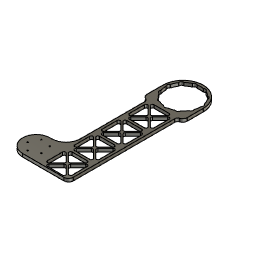
Arm section 1_v10 (Autodesk Fusion 360 design; units mm, degrees)
Autodesk Fusion 360 part; units mm, degrees
sketch "Sketch2" plane through (0, 0, 0) normal (0, 0, 1) x (1, 0, 0)
  line L0 (0, 0) -> (96, 0)
  line L1 (96, 0) -> (96, 96)
  line L2 (96, 96) -> (0, 96)
  line L3 (0, 96) -> (0, 0)
  line L4 (8, 8) -> (88, 8)
  line L5 (88, 8) -> (88, 88)
  line L6 (88, 88) -> (8, 88)
  line L7 (8, 88) -> (8, 8)
  line L8 (8, 88) -> (88, 8) construction
  line L9 (8, 8) -> (88, 88) construction
  line L10 (6.2322, 86.2322) -> (86.2322, 6.2322)
  line L11 (9.7678, 89.7678) -> (89.7678, 9.7678)
  line L12 (9.7678, 6.2322) -> (89.7678, 86.2322)
  line L13 (6.2322, 9.7678) -> (86.2322, 89.7678)
  dimension "d17" = 96
  dimension "d18" = 96
  dimension "d19" = 80
  dimension "d20" = 80
  dimension "d21" = 8
  dimension "d22" = 8
  dimension "d23" = 2.5
  dimension "d24" = -2.5
  dimension "d25" = 2.5
  dimension "d26" = -2.5
  constraint horizontal L0
  constraint vertical L1
  constraint horizontal L2
  constraint vertical L3
  constraint coincident L0.start L3.end
  constraint horizontal L4
  constraint vertical L5
  constraint horizontal L6
  constraint vertical L7
  measures "d17" distance of L0.start L0.end
  measures "d18" distance of L0.start L2.end
  measures "d19" distance of L4.start L4.end
  measures "d20" distance of L4.start L6.end
  measures "d21" distance of L3 L7
  measures "d22" distance of L0 L4
extrude "Extrude2" add sketch "Sketch2" along normal blind 20 contours L0 L1 L2 L3 | L4 L7 L10 L12 L13 | L4 L5 L10 L11 L12 | L10 L11 L12 L13 | L6 L7 L10 L11 L13 | L5 L6 L11 L12 L13 makes body 1
fillet "Fillet1" radius 5 4 edges at (48, 44.4645, 10) (44.4645, 48, 10) (48, 51.5355, 10) (51.5355, 48, 10) on bodies 1
fillet "Fillet1" radius 5 8 edges at (8, 11.5355, 10) (8, 84.4645, 10) (11.5355, 88, 10) (84.4645, 88, 10) (88, 84.4645, 10) (88, 11.5355, 10) (84.4645, 8, 10) (11.5355, 8, 10) on bodies 1
extrude "Extrude3" cut 1 faces at (64, 96, 6.6667) along direction (0, -1, 0) blind 4 on bodies 1 bodies 1
extrude "Extrude4" cut 1 faces at (32, 0, 6.6667) along direction (0, 1, 0) blind 4 on bodies 1 bodies 1
pattern_linear "R-Pattern1" count 4 spacing 88 along (0, 1, 0) of bodies 1 makes body 2 at (93.3333, 127.8689, 0) makes body 3 at (93.3333, 232.1311, 0) makes body 4 at (93.3333, 320.1311, 0)
combine "Combine1" operation add target body 1 tool bodies 2 3 4
sketch "Sketch3" plane through (0, 0, 0) normal (0, 0, 1) x (1, 0, 0)
  line L0 (0, 356) -> (0, 4)
  line L1 (0, 4) -> (-96, 4)
  line L2 (-96, 4) -> (-96, 92)
  line L3 (-96, 92) -> (0, 92)
  line L4 (0, 92) -> (0, 4)
  line L5 (0, 92) -> (-96, 4) construction
  line L6 (-96, 92) -> (0, 4) construction
  circle A0 centre (-48, 48) radius 28 construction
  circle A1 centre (-75.6627, 43.6673) radius 2
  circle A2 centre (-52.4276, 20.3523) radius 2
  circle A3 centre (-23.0737, 35.2455) radius 2
  circle A4 centre (-28.1671, 67.765) radius 2
  circle A5 centre (-60.6689, 72.9699) radius 2
  circle A6 centre (-35.3311, 23.0301) radius 2
  circle A7 centre (-67.8329, 28.235) radius 2
  circle A8 centre (-72.9263, 60.7545) radius 2
  circle A9 centre (-43.5724, 75.6477) radius 2
  circle A10 centre (-20.3373, 52.3327) radius 2
  dimension "d44" = 96
  dimension "d45" = 88
  dimension "d46" = 56
  dimension "d47" = 4
  dimension "d49" = 360
  dimension "d145" = 360
  constraint horizontal L1
  constraint vertical L2
  constraint horizontal L3
  constraint vertical L4
  constraint coincident L0.end L1.start
  constraint midpoint L5 A0.centre
  constraint coincident A0 A1.centre
  measures "d44" distance of L0.end L1.end
  measures "d45" distance of L0.end L3.end
  measures "d46" diameter of A0
  measures "d47" diameter of A1
extrude "Extrude5" add sketch "Sketch3" along normal blind 20 bodies 1
fillet "Fillet2" radius 44 2 edges at (-96, 92, 10) (-96, 4, 10) on bodies 1
fillet "Fillet3" radius 46 1 edges at (0, 92, 10) on bodies 1
fillet "Fillet4" radius 15 1 edges at (96, 4, 10) on bodies 1
extrude "Extrude7" cut 1 faces at (-0.7791, 49.4442, 20) along direction (0, 0, -1) blind 10 on bodies 1 bodies 1
sketch "Sketch6" plane through (0, 0, 0) normal (0, 0, 1) x (1, 0, 0)
  circle A0 centre (48, 436) radius 65
  circle A1 centre (48, 436) radius 80
  line L0 (0, 356) -> (96, 356)
  line L1 (96, 356) -> (128, 356) construction
  line L2 (128, 356) -> (-32, 356)
  line L3 (-32, 356) -> (-32, 516)
  line L4 (-32, 516) -> (128, 516)
  line L5 (128, 516) -> (128, 356)
  point P0 (96, 356)
  point P1 (0, 356)
  dimension "d78" = 130
  dimension "d81" = 160
  dimension "d89" = 80
  dimension "d90" = 32
  dimension "d91" = 160
  dimension "d92" = 160
  constraint concentric A0 A1
  constraint coincident P0 L0.end
  constraint parallel L0 L1
  constraint horizontal L2
  constraint vertical L3
  constraint horizontal L4
  constraint vertical L5
  measures "d78" diameter of A0
  measures "d81" diameter of A1
  measures "d89" distance of A0.centre L0
  measures "d90" distance of P0 L1.end
  measures "d91" distance of L1.end L2.end
  measures "d92" distance of L1.end L4.end
extrude "Extrude8" add sketch "Sketch6" along normal blind 10 contours A1 | A1 L0 L2 L5 | A1 L0 L2 L3 bodies 1
fillet "Fillet6" radius 15 2 edges at (96, 356, 5) (0, 356, 5) on bodies 1
fillet "Fillet6" radius 15 2 edges at (-32, 356, 5) (128, 356, 5) on bodies 1
sketch "Sketch7" plane through (0, 0, 10) normal (0, 0, 1) x (-1, 0, 0)
  arc A0 (-113, -356) -> (-128, -371) centre (-113, -371) ccw
  line L0 (-128, -371) -> (-128, -436)
  arc A1 (-128, -436) -> (32, -436) centre (-48, -436) ccw
  line L1 (32, -436) -> (32, -371)
  arc A2 (32, -371) -> (17, -356) centre (17, -371) ccw
  line L2 (17, -356) -> (15, -356)
  arc A3 (0, -341) -> (15, -356) centre (15, -341) ccw
  line L3 (0, -341) -> (0, -138)
  arc A4 (46, -92) -> (0, -138) centre (46, -138) ccw
  line L4 (46, -92) -> (52, -92)
  arc A5 (52, -92) -> (52, -4) centre (52, -48) ccw
  line L5 (52, -4) -> (-81, -4)
  arc A6 (-81, -4) -> (-96, -19) centre (-81, -19) ccw
  line L6 (-96, -19) -> (-96, -341)
  arc A7 (-111, -356) -> (-96, -341) centre (-111, -341) ccw
  line L7 (-111, -356) -> (-113, -356)
  circle A8 centre (-48, -436) radius 65
  circle A9 centre (23.0737, -35.2455) radius 2
  circle A10 centre (75.6627, -43.6673) radius 2
  circle A11 centre (52.4276, -20.3523) radius 2
  circle A12 centre (60.6689, -72.9699) radius 2
  circle A13 centre (28.1671, -67.765) radius 2
  line L8 (-20.0711, -280.5355) -> (-44.4645, -304.9289)
  arc A14 (-51.5355, -304.9289) -> (-44.4645, -304.9289) centre (-48, -301.3934) ccw
  line L9 (-51.5355, -304.9289) -> (-75.9289, -280.5355)
  arc A15 (-72.3934, -272) -> (-75.9289, -280.5355) centre (-72.3934, -277) ccw
  line L10 (-72.3934, -272) -> (-23.6066, -272)
  arc A16 (-20.0711, -280.5355) -> (-23.6066, -272) centre (-23.6066, -277) ccw
  line L11 (-79.4645, -284.0711) -> (-55.0711, -308.4645)
  arc A17 (-55.0711, -315.5355) -> (-55.0711, -308.4645) centre (-58.6066, -312) ccw
  line L12 (-55.0711, -315.5355) -> (-79.4645, -339.9289)
  arc A18 (-88, -336.3934) -> (-79.4645, -339.9289) centre (-83, -336.3934) ccw
  line L13 (-88, -336.3934) -> (-88, -287.6066)
  arc A19 (-79.4645, -284.0711) -> (-88, -287.6066) centre (-83, -287.6066) ccw
  line L14 (-8, -287.6066) -> (-8, -336.3934)
  arc A20 (-16.5355, -339.9289) -> (-8, -336.3934) centre (-13, -336.3934) ccw
  line L15 (-16.5355, -339.9289) -> (-40.9289, -315.5355)
  arc A21 (-40.9289, -308.4645) -> (-40.9289, -315.5355) centre (-37.3934, -312) ccw
  line L16 (-40.9289, -308.4645) -> (-16.5355, -284.0711)
  arc A22 (-8, -287.6066) -> (-16.5355, -284.0711) centre (-13, -287.6066) ccw
  line L17 (-44.4645, -319.0711) -> (-20.0711, -343.4645)
  arc A23 (-23.6066, -352) -> (-20.0711, -343.4645) centre (-23.6066, -347) ccw
  line L18 (-23.6066, -352) -> (-72.3934, -352)
  arc A24 (-75.9289, -343.4645) -> (-72.3934, -352) centre (-72.3934, -347) ccw
  line L19 (-75.9289, -343.4645) -> (-51.5355, -319.0711)
  arc A25 (-44.4645, -319.0711) -> (-51.5355, -319.0711) centre (-48, -322.6066) ccw
  line L20 (-20.0711, -192.5355) -> (-44.4645, -216.9289)
  arc A26 (-51.5355, -216.9289) -> (-44.4645, -216.9289) centre (-48, -213.3934) ccw
  line L21 (-51.5355, -216.9289) -> (-75.9289, -192.5355)
  arc A27 (-72.3934, -184) -> (-75.9289, -192.5355) centre (-72.3934, -189) ccw
  line L22 (-72.3934, -184) -> (-23.6066, -184)
  arc A28 (-20.0711, -192.5355) -> (-23.6066, -184) centre (-23.6066, -189) ccw
  line L23 (-79.4645, -196.0711) -> (-55.0711, -220.4645)
  arc A29 (-55.0711, -227.5355) -> (-55.0711, -220.4645) centre (-58.6066, -224) ccw
  line L24 (-55.0711, -227.5355) -> (-79.4645, -251.9289)
  arc A30 (-88, -248.3934) -> (-79.4645, -251.9289) centre (-83, -248.3934) ccw
  line L25 (-88, -248.3934) -> (-88, -199.6066)
  arc A31 (-79.4645, -196.0711) -> (-88, -199.6066) centre (-83, -199.6066) ccw
  line L26 (-8, -199.6066) -> (-8, -248.3934)
  arc A32 (-16.5355, -251.9289) -> (-8, -248.3934) centre (-13, -248.3934) ccw
  line L27 (-16.5355, -251.9289) -> (-40.9289, -227.5355)
  arc A33 (-40.9289, -220.4645) -> (-40.9289, -227.5355) centre (-37.3934, -224) ccw
  line L28 (-40.9289, -220.4645) -> (-16.5355, -196.0711)
  arc A34 (-8, -199.6066) -> (-16.5355, -196.0711) centre (-13, -199.6066) ccw
  line L29 (-44.4645, -231.0711) -> (-20.0711, -255.4645)
  arc A35 (-23.6066, -264) -> (-20.0711, -255.4645) centre (-23.6066, -259) ccw
  line L30 (-23.6066, -264) -> (-72.3934, -264)
  arc A36 (-75.9289, -255.4645) -> (-72.3934, -264) centre (-72.3934, -259) ccw
  line L31 (-75.9289, -255.4645) -> (-51.5355, -231.0711)
  arc A37 (-44.4645, -231.0711) -> (-51.5355, -231.0711) centre (-48, -234.6066) ccw
  line L32 (-20.0711, -104.5355) -> (-44.4645, -128.9289)
  arc A38 (-51.5355, -128.9289) -> (-44.4645, -128.9289) centre (-48, -125.3934) ccw
  line L33 (-51.5355, -128.9289) -> (-75.9289, -104.5355)
  arc A39 (-72.3934, -96) -> (-75.9289, -104.5355) centre (-72.3934, -101) ccw
  line L34 (-72.3934, -96) -> (-23.6066, -96)
  arc A40 (-20.0711, -104.5355) -> (-23.6066, -96) centre (-23.6066, -101) ccw
  line L35 (-79.4645, -108.0711) -> (-55.0711, -132.4645)
  arc A41 (-55.0711, -139.5355) -> (-55.0711, -132.4645) centre (-58.6066, -136) ccw
  line L36 (-55.0711, -139.5355) -> (-79.4645, -163.9289)
  arc A42 (-88, -160.3934) -> (-79.4645, -163.9289) centre (-83, -160.3934) ccw
  line L37 (-88, -160.3934) -> (-88, -111.6066)
  arc A43 (-79.4645, -108.0711) -> (-88, -111.6066) centre (-83, -111.6066) ccw
  line L38 (-8, -111.6066) -> (-8, -160.3934)
  arc A44 (-16.5355, -163.9289) -> (-8, -160.3934) centre (-13, -160.3934) ccw
  line L39 (-16.5355, -163.9289) -> (-40.9289, -139.5355)
  arc A45 (-40.9289, -132.4645) -> (-40.9289, -139.5355) centre (-37.3934, -136) ccw
  line L40 (-40.9289, -132.4645) -> (-16.5355, -108.0711)
  arc A46 (-8, -111.6066) -> (-16.5355, -108.0711) centre (-13, -111.6066) ccw
  line L41 (-44.4645, -143.0711) -> (-20.0711, -167.4645)
  arc A47 (-23.6066, -176) -> (-20.0711, -167.4645) centre (-23.6066, -171) ccw
  line L42 (-23.6066, -176) -> (-72.3934, -176)
  arc A48 (-75.9289, -167.4645) -> (-72.3934, -176) centre (-72.3934, -171) ccw
  line L43 (-75.9289, -167.4645) -> (-51.5355, -143.0711)
  arc A49 (-44.4645, -143.0711) -> (-51.5355, -143.0711) centre (-48, -146.6066) ccw
  line L44 (-44.4645, -55.0711) -> (-20.0711, -79.4645)
  arc A50 (-23.6066, -88) -> (-20.0711, -79.4645) centre (-23.6066, -83) ccw
  line L45 (-23.6066, -88) -> (-72.3934, -88)
  arc A51 (-75.9289, -79.4645) -> (-72.3934, -88) centre (-72.3934, -83) ccw
  line L46 (-75.9289, -79.4645) -> (-51.5355, -55.0711)
  arc A52 (-44.4645, -55.0711) -> (-51.5355, -55.0711) centre (-48, -58.6066) ccw
  line L47 (-8, -23.6066) -> (-8, -72.3934)
  arc A53 (-16.5355, -75.9289) -> (-8, -72.3934) centre (-13, -72.3934) ccw
  line L48 (-16.5355, -75.9289) -> (-40.9289, -51.5355)
  arc A54 (-40.9289, -44.4645) -> (-40.9289, -51.5355) centre (-37.3934, -48) ccw
  line L49 (-40.9289, -44.4645) -> (-16.5355, -20.0711)
  arc A55 (-8, -23.6066) -> (-16.5355, -20.0711) centre (-13, -23.6066) ccw
  line L50 (-79.4645, -20.0711) -> (-55.0711, -44.4645)
  arc A56 (-55.0711, -51.5355) -> (-55.0711, -44.4645) centre (-58.6066, -48) ccw
  line L51 (-55.0711, -51.5355) -> (-79.4645, -75.9289)
  arc A57 (-88, -72.3934) -> (-79.4645, -75.9289) centre (-83, -72.3934) ccw
  line L52 (-88, -72.3934) -> (-88, -23.6066)
  arc A58 (-79.4645, -20.0711) -> (-88, -23.6066) centre (-83, -23.6066) ccw
  line L53 (-20.0711, -16.5355) -> (-44.4645, -40.9289)
  arc A59 (-51.5355, -40.9289) -> (-44.4645, -40.9289) centre (-48, -37.3934) ccw
  line L54 (-51.5355, -40.9289) -> (-75.9289, -16.5355)
  arc A60 (-72.3934, -8) -> (-75.9289, -16.5355) centre (-72.3934, -13) ccw
  line L55 (-72.3934, -8) -> (-23.6066, -8)
  arc A61 (-20.0711, -16.5355) -> (-23.6066, -8) centre (-23.6066, -13) ccw
  circle A62 through (-94.852, -379.4242, 0.398) (-96.952, -378.2118, 0.398) (-96.952, -380.6366, 0.398)
  line L56 (-48, -436, -15) -> (-48, -436, 5)
  circle A63 centre (72.9263, -60.7545) radius 2
  circle A64 centre (35.3311, -23.0301) radius 2
  circle A65 centre (20.3373, -52.3327) radius 2
  circle A66 centre (43.5724, -75.6477) radius 2
  circle A67 centre (67.8329, -28.235) radius 2
  dimension "d97" = 2.8
  dimension "d100" = 74.5
extrude "Extrude9" cut sketch "Sketch7" against normal blind 36 contours A62 in plane through (0, 0, 10.398) normal (0, 0, 1) bodies 1
pattern_circular "C-Pattern1" count 3 over 360 about axis through (48, 436, -5) along (0, 0, 1) of "Extrude9"
sketch "Sketch8" plane through (0, 0, 10) normal (0, 0, 1) x (-1, 0, 0)
  circle A0 centre (25.1221, -422.5005) radius 1.4
  circle A1 centre (-72.8701, -506.0753) radius 1.4
  circle A2 centre (-96.252, -379.4242) radius 1.4
  arc A3 (-113, -356) -> (-128, -371) centre (-113, -371) ccw
  line L0 (-128, -371) -> (-128, -436)
  arc A4 (-128, -436) -> (32, -436) centre (-48, -436) ccw
  line L1 (32, -436) -> (32, -371)
  arc A5 (32, -371) -> (17, -356) centre (17, -371) ccw
  line L2 (17, -356) -> (15, -356)
  arc A6 (0, -341) -> (15, -356) centre (15, -341) ccw
  line L3 (0, -341) -> (0, -138)
  arc A7 (46, -92) -> (0, -138) centre (46, -138) ccw
  line L4 (46, -92) -> (52, -92)
  arc A8 (52, -92) -> (52, -4) centre (52, -48) ccw
  line L5 (52, -4) -> (-81, -4)
  arc A9 (-81, -4) -> (-96, -19) centre (-81, -19) ccw
  line L6 (-96, -19) -> (-96, -341)
  arc A10 (-111, -356) -> (-96, -341) centre (-111, -341) ccw
  line L7 (-111, -356) -> (-113, -356)
  circle A11 centre (-48, -436) radius 65
  circle A12 centre (23.0737, -35.2455) radius 2
  circle A13 centre (75.6627, -43.6673) radius 2
  circle A14 centre (52.4276, -20.3523) radius 2
  circle A15 centre (60.6689, -72.9699) radius 2
  circle A16 centre (28.1671, -67.765) radius 2
  line L8 (-20.0711, -280.5355) -> (-44.4645, -304.9289)
  arc A17 (-51.5355, -304.9289) -> (-44.4645, -304.9289) centre (-48, -301.3934) ccw
  line L9 (-51.5355, -304.9289) -> (-75.9289, -280.5355)
  arc A18 (-72.3934, -272) -> (-75.9289, -280.5355) centre (-72.3934, -277) ccw
  line L10 (-72.3934, -272) -> (-23.6066, -272)
  arc A19 (-20.0711, -280.5355) -> (-23.6066, -272) centre (-23.6066, -277) ccw
  line L11 (-79.4645, -284.0711) -> (-55.0711, -308.4645)
  arc A20 (-55.0711, -315.5355) -> (-55.0711, -308.4645) centre (-58.6066, -312) ccw
  line L12 (-55.0711, -315.5355) -> (-79.4645, -339.9289)
  arc A21 (-88, -336.3934) -> (-79.4645, -339.9289) centre (-83, -336.3934) ccw
  line L13 (-88, -336.3934) -> (-88, -287.6066)
  arc A22 (-79.4645, -284.0711) -> (-88, -287.6066) centre (-83, -287.6066) ccw
  line L14 (-8, -287.6066) -> (-8, -336.3934)
  arc A23 (-16.5355, -339.9289) -> (-8, -336.3934) centre (-13, -336.3934) ccw
  line L15 (-16.5355, -339.9289) -> (-40.9289, -315.5355)
  arc A24 (-40.9289, -308.4645) -> (-40.9289, -315.5355) centre (-37.3934, -312) ccw
  line L16 (-40.9289, -308.4645) -> (-16.5355, -284.0711)
  arc A25 (-8, -287.6066) -> (-16.5355, -284.0711) centre (-13, -287.6066) ccw
  line L17 (-44.4645, -319.0711) -> (-20.0711, -343.4645)
  arc A26 (-23.6066, -352) -> (-20.0711, -343.4645) centre (-23.6066, -347) ccw
  line L18 (-23.6066, -352) -> (-72.3934, -352)
  arc A27 (-75.9289, -343.4645) -> (-72.3934, -352) centre (-72.3934, -347) ccw
  line L19 (-75.9289, -343.4645) -> (-51.5355, -319.0711)
  arc A28 (-44.4645, -319.0711) -> (-51.5355, -319.0711) centre (-48, -322.6066) ccw
  line L20 (-20.0711, -192.5355) -> (-44.4645, -216.9289)
  arc A29 (-51.5355, -216.9289) -> (-44.4645, -216.9289) centre (-48, -213.3934) ccw
  line L21 (-51.5355, -216.9289) -> (-75.9289, -192.5355)
  arc A30 (-72.3934, -184) -> (-75.9289, -192.5355) centre (-72.3934, -189) ccw
  line L22 (-72.3934, -184) -> (-23.6066, -184)
  arc A31 (-20.0711, -192.5355) -> (-23.6066, -184) centre (-23.6066, -189) ccw
  line L23 (-79.4645, -196.0711) -> (-55.0711, -220.4645)
  arc A32 (-55.0711, -227.5355) -> (-55.0711, -220.4645) centre (-58.6066, -224) ccw
  line L24 (-55.0711, -227.5355) -> (-79.4645, -251.9289)
  arc A33 (-88, -248.3934) -> (-79.4645, -251.9289) centre (-83, -248.3934) ccw
  line L25 (-88, -248.3934) -> (-88, -199.6066)
  arc A34 (-79.4645, -196.0711) -> (-88, -199.6066) centre (-83, -199.6066) ccw
  line L26 (-8, -199.6066) -> (-8, -248.3934)
  arc A35 (-16.5355, -251.9289) -> (-8, -248.3934) centre (-13, -248.3934) ccw
  line L27 (-16.5355, -251.9289) -> (-40.9289, -227.5355)
  arc A36 (-40.9289, -220.4645) -> (-40.9289, -227.5355) centre (-37.3934, -224) ccw
  line L28 (-40.9289, -220.4645) -> (-16.5355, -196.0711)
  arc A37 (-8, -199.6066) -> (-16.5355, -196.0711) centre (-13, -199.6066) ccw
  line L29 (-44.4645, -231.0711) -> (-20.0711, -255.4645)
  arc A38 (-23.6066, -264) -> (-20.0711, -255.4645) centre (-23.6066, -259) ccw
  line L30 (-23.6066, -264) -> (-72.3934, -264)
  arc A39 (-75.9289, -255.4645) -> (-72.3934, -264) centre (-72.3934, -259) ccw
  line L31 (-75.9289, -255.4645) -> (-51.5355, -231.0711)
  arc A40 (-44.4645, -231.0711) -> (-51.5355, -231.0711) centre (-48, -234.6066) ccw
  line L32 (-20.0711, -104.5355) -> (-44.4645, -128.9289)
  arc A41 (-51.5355, -128.9289) -> (-44.4645, -128.9289) centre (-48, -125.3934) ccw
  line L33 (-51.5355, -128.9289) -> (-75.9289, -104.5355)
  arc A42 (-72.3934, -96) -> (-75.9289, -104.5355) centre (-72.3934, -101) ccw
  line L34 (-72.3934, -96) -> (-23.6066, -96)
  arc A43 (-20.0711, -104.5355) -> (-23.6066, -96) centre (-23.6066, -101) ccw
  line L35 (-79.4645, -108.0711) -> (-55.0711, -132.4645)
  arc A44 (-55.0711, -139.5355) -> (-55.0711, -132.4645) centre (-58.6066, -136) ccw
  line L36 (-55.0711, -139.5355) -> (-79.4645, -163.9289)
  arc A45 (-88, -160.3934) -> (-79.4645, -163.9289) centre (-83, -160.3934) ccw
  line L37 (-88, -160.3934) -> (-88, -111.6066)
  arc A46 (-79.4645, -108.0711) -> (-88, -111.6066) centre (-83, -111.6066) ccw
  line L38 (-8, -111.6066) -> (-8, -160.3934)
  arc A47 (-16.5355, -163.9289) -> (-8, -160.3934) centre (-13, -160.3934) ccw
  line L39 (-16.5355, -163.9289) -> (-40.9289, -139.5355)
  arc A48 (-40.9289, -132.4645) -> (-40.9289, -139.5355) centre (-37.3934, -136) ccw
  line L40 (-40.9289, -132.4645) -> (-16.5355, -108.0711)
  arc A49 (-8, -111.6066) -> (-16.5355, -108.0711) centre (-13, -111.6066) ccw
  line L41 (-44.4645, -143.0711) -> (-20.0711, -167.4645)
  arc A50 (-23.6066, -176) -> (-20.0711, -167.4645) centre (-23.6066, -171) ccw
  line L42 (-23.6066, -176) -> (-72.3934, -176)
  arc A51 (-75.9289, -167.4645) -> (-72.3934, -176) centre (-72.3934, -171) ccw
  line L43 (-75.9289, -167.4645) -> (-51.5355, -143.0711)
  arc A52 (-44.4645, -143.0711) -> (-51.5355, -143.0711) centre (-48, -146.6066) ccw
  line L44 (-44.4645, -55.0711) -> (-20.0711, -79.4645)
  arc A53 (-23.6066, -88) -> (-20.0711, -79.4645) centre (-23.6066, -83) ccw
  line L45 (-23.6066, -88) -> (-72.3934, -88)
  arc A54 (-75.9289, -79.4645) -> (-72.3934, -88) centre (-72.3934, -83) ccw
  line L46 (-75.9289, -79.4645) -> (-51.5355, -55.0711)
  arc A55 (-44.4645, -55.0711) -> (-51.5355, -55.0711) centre (-48, -58.6066) ccw
  line L47 (-8, -23.6066) -> (-8, -72.3934)
  arc A56 (-16.5355, -75.9289) -> (-8, -72.3934) centre (-13, -72.3934) ccw
  line L48 (-16.5355, -75.9289) -> (-40.9289, -51.5355)
  arc A57 (-40.9289, -44.4645) -> (-40.9289, -51.5355) centre (-37.3934, -48) ccw
  line L49 (-40.9289, -44.4645) -> (-16.5355, -20.0711)
  arc A58 (-8, -23.6066) -> (-16.5355, -20.0711) centre (-13, -23.6066) ccw
  line L50 (-79.4645, -20.0711) -> (-55.0711, -44.4645)
  arc A59 (-55.0711, -51.5355) -> (-55.0711, -44.4645) centre (-58.6066, -48) ccw
  line L51 (-55.0711, -51.5355) -> (-79.4645, -75.9289)
  arc A60 (-88, -72.3934) -> (-79.4645, -75.9289) centre (-83, -72.3934) ccw
  line L52 (-88, -72.3934) -> (-88, -23.6066)
  arc A61 (-79.4645, -20.0711) -> (-88, -23.6066) centre (-83, -23.6066) ccw
  line L53 (-20.0711, -16.5355) -> (-44.4645, -40.9289)
  arc A62 (-51.5355, -40.9289) -> (-44.4645, -40.9289) centre (-48, -37.3934) ccw
  line L54 (-51.5355, -40.9289) -> (-75.9289, -16.5355)
  arc A63 (-72.3934, -8) -> (-75.9289, -16.5355) centre (-72.3934, -13) ccw
  line L55 (-72.3934, -8) -> (-23.6066, -8)
  arc A64 (-20.0711, -16.5355) -> (-23.6066, -8) centre (-23.6066, -13) ccw
  circle A65 centre (-96, -180) radius 18
  circle A66 centre (-96, -180) radius 12.5
  circle A67 centre (-89.75, -169.1747) radius 1.5
  circle A68 centre (-85.1747, -173.75) radius 1.5
  line L56 (-89.75, -169.1747) -> (-96, -180) construction
  line L57 (-85.1747, -173.75) -> (-96, -180) construction
  circle A69 centre (-85.1747, -186.25) radius 1.5
  circle A70 centre (-89.75, -190.8253) radius 1.5
  line L58 (-96, -180) -> (-85.1747, -186.25) construction
  line L59 (-96, -180) -> (-89.75, -190.8253) construction
  line L60 (-96, -162) -> (-96, -198)
  circle A71 centre (72.9263, -60.7545) radius 2
  circle A72 centre (35.3311, -23.0301) radius 2
  circle A73 centre (20.3373, -52.3327) radius 2
  circle A74 centre (43.5724, -75.6477) radius 2
  circle A75 centre (67.8329, -28.235) radius 2
  dimension "d105" = 36
  dimension "d106" = 25
  dimension "d107" = 3
  dimension "d108" = 3
  dimension "d109" = 150
  dimension "d110" = 60
  dimension "d111" = 3
  dimension "d112" = 3
  dimension "d113" = 60
  dimension "d114" = 30
  constraint midpoint L6 A65.centre
  constraint concentric A65 A66
  constraint coincident A66 A67.centre
  constraint coincident A66 A68.centre
  constraint coincident A67.centre L56.start
  constraint coincident A65.centre A66.centre
  constraint coincident A68.centre L57.start
  constraint coincident A66 A69.centre
  constraint coincident A66 A70.centre
  constraint coincident A69.centre L58.end
  constraint coincident A70.centre L59.end
  constraint coincident A65 L60.start
  constraint coincident L6 L60.start
  constraint coincident A65 L60.end
  constraint coincident L6 L60.end
  measures "d105" diameter of A65
  measures "d106" diameter of A66
  measures "d107" diameter of A67
  measures "d108" diameter of A68
  measures "d109" angle of L6 L56
  measures "d110" angle of L6 L57
  measures "d111" diameter of A69
  measures "d112" diameter of A70
  measures "d113" angle of L6 L58
  measures "d114" angle of L6 L59
extrude "Extrude10" add sketch "Sketch8" along normal blind 4 separate body contours L6 A65 A66 A67 A68 A69 A70 L60 | L6 A66 A67 A68 A69 A70 L60 makes body 5
ref_plane "WorkPlane2" through (-16, 356, 5) normal (0, -1, 0) x (1, 0, 0)
split "Split1" by plane through (-16, 356, 5) normal (0, -1, 0) bodies 1 makes body 6 at (-0.7791, 49.4442, 0)
ref_plane "WorkPlane3" through (48, 180, 5) normal (0, 1, 0) x (-1, 0, 0)
split "Split2" by plane through (48, 180, 5) normal (0, 1, 0) bodies 6 makes body 7 at (2.6667, 256.4645, 0)
extrude "Extrude11" cut sketch "Sketch8" against normal blind 13 contours A66 A70 | A66 A70 | A66 A67 | A66 A67 | A66 A69 | A66 A69 | A66 A68 | A66 A68 bodies 6 7
ref_plane "WorkPlane4" through (48, 260.5, 5) normal (1, 0, 0) x (0, 1, 0)
mirror "Mirror3" about plane through (48, 260.5, 5) normal (1, 0, 0) of "Extrude11"
ref_plane "WorkPlane5" through (48, 268, 5) normal (0, 1, 0) x (-1, 0, 0)
mirror "Mirror4" about plane through (48, 268, 5) normal (0, 1, 0) of "Extrude11", "Mirror3"
sketch "Sketch10" plane through (0, 0, 10) normal (0, 0, 1) x (-1, 0, 0)
  line L0 (-96, -341) -> (-96, -180) construction
  line L1 (-113, -356) -> (17, -356) construction
  line L2 (-96, -335.0263) -> (-96, -356) construction
  circle A0 centre (-96, -356) radius 12.5 construction
  circle A1 centre (-85.1747, -362.25) radius 1.5
  circle A2 centre (-89.75, -366.8253) radius 1.5
  line L3 (-85.1747, -362.25) -> (-96, -356) construction
  line L4 (-89.75, -366.8253) -> (-96, -356) construction
  dimension "d126" = 25
  dimension "d127" = 3
  dimension "d128" = 3
  dimension "d129" = 30
  dimension "d130" = 60
  constraint vertical L2
  constraint coincident L0 L2.start
  constraint coincident L1 L2.end
  constraint coincident L2.end A0.centre
  constraint coincident A0 A1.centre
  constraint coincident A0 A2.centre
  constraint coincident A1.centre L3.start
  constraint coincident A2.centre L4.start
  measures "d126" diameter of A0
  measures "d127" diameter of A1
  measures "d128" diameter of A2
  measures "d129" angle of L1 L3
  measures "d130" angle of L1 L4
extrude "Extrude12" cut sketch "Sketch10" against normal blind 20 bodies 1
mirror "Mirror6" about plane through (48, 260.5, 5) normal (1, 0, 0) of "Extrude12"
copy_body "CopyPasteBodies1" bodies 1 makes body 8
move_body "Move1" bodies 8 to x (1, 0, 0) y (0, 1, 0) z (0, 0, 1) at (180, 0, 0)
move_face "OffsetFaces1" offset 25.5 1 faces at (163.323, 429.5281, 3.3333) on bodies 8
sketch "Sketch12" plane through (0, 0, 10) normal (0, 0, 1) x (-1, 0, 0)
  circle A0 centre (-190.8253, -362.25) radius 1.5
  circle A1 centre (-186.25, -366.8253) radius 1.5
  circle A2 centre (-265.1747, -362.25) radius 1.5
  circle A3 centre (-269.75, -366.8253) radius 1.5
  line L0 (-163, -356) -> (-293, -356)
  arc A4 (-293, -356) -> (-308, -371) centre (-293, -371) ccw
  line L1 (-308, -371) -> (-308, -436)
  arc A5 (-308, -436) -> (-148, -436) centre (-228, -436) ccw
  line L2 (-148, -436) -> (-148, -371)
  arc A6 (-148, -371) -> (-163, -356) centre (-163, -371) ccw
  circle A7 centre (-154.8779, -422.5005) radius 1.4
  circle A8 centre (-252.8701, -506.0753) radius 1.4
  circle A9 centre (-276.252, -379.4242) radius 1.4
  circle A10 centre (-228, -436) radius 39.5
  circle A11 centre (-228, -436) radius 42.75
  dimension "d147" = 85.5
  constraint concentric A5 A11
  measures "d147" diameter of A11
extrude "Extrude14" cut sketch "Sketch12" against normal blind 8 contours A11 bodies 8
copy_body "CopyPasteBodies2" bodies 5 makes body 9
move_body "Move2" bodies 9 to x (1, 0, 0) y (0, 1, 0) z (0, 0, 1) at (60, 0, 0)
extrude "Extrude15" add 1 faces at (142.4689, 180, 14) along direction (0, 0, 1) blind 37 on bodies 9 bodies 9
equation "d81 = gearboxDia + 30 mm"
equation "gearboxDia = 130 mm"
equation "d89 = gearboxDia / 2 + 15 mm"
equation "d90 = ( gearboxDia - 96 mm ) / 2 + 15 mm"
equation "d91 = gearboxDia + 30 mm"
equation "d92 = gearboxDia + 30 mm"
named bodies: "Arm Elbow", "Brace", "Sholder arm", "Bone", "Arm Elbow (1)", "Brace (1)"
